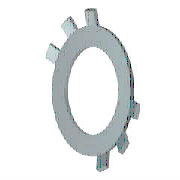
# Autodesk Inventor part: 垫圈 GB 858 30
Saved by Autodesk Inventor 2020 (Build 240168000, 168)
## iProperties
Created: 2019-01-21
Part Number: 垫圈 GB 858 30
Material: 钢，软
Description: 圆螺母的止动垫圈
Document SubType Name: Modeling
Standard: GB/T 858-1988
Designer: dell
Standard Revision: 1988
Standards Organization: GB
Language: zh-CN
Size Designation: 30 x 40
Categories: <MemberInstance><Categories><Category DisplayName="轴用零件" InternalName="7f7aeb1f-a693-4053-b835-cee3144e0d98" Mnemonic="SHFT"><Category DisplayName="止动垫圈" InternalName="196297a3-bbf2-4c62-a426-6f1b43e49a92" Mnemonic="STWRDBRCMP"><CategoryParameter DisplayName="接触区域直径" InternalName="2e92645a-023d-4b6f-85cb-aa6579b07711" Mnemonic="conarea"/><CategoryParameter DisplayName="沟槽高度" InternalName="459e1daf-c3a8-40cb-aa85-2a4675385d1b" Mnemonic="grvheig"/><CategoryParameter DisplayName="厚度" InternalName="5f8ad5cd-5310-44ac-8ee3-8a10cbe3cc2a" Mnemonic="thick"/><CategoryParameter DisplayName="轴直径" InternalName="a5cdae98-95ea-47ec-9880-d704d388e74c" Mnemonic="shaftdia"/></Category></Category><Category DisplayName="数据类型" InternalName="23b78d0f-2648-40c6-8793-ca6db495c9e8" Mnemonic="DATATYPE"><CategoryParameter DisplayName="显示名" InternalName="05415f3d-3907-474b-a020-eb9d644f4cf3" Mnemonic="DISPLAYNAME"/><CategoryParameter DisplayName="标准" InternalName="0c0a119c-1e12-4c84-803f-101930972f5e" Mnemonic="STANDARD"/><CategoryParameter DisplayName="描述" InternalName="13903e3d-64b1-4950-80da-f627842ea37f" Mnemonic="DESCRIPTION"/><CategoryParameter DisplayName="规格" InternalName="2675968c-4ce5-49e0-a4f5-552d29089031" Mnemonic="DESIGNATION"/><CategoryParameter DisplayName="默认列" InternalName="2af9ec52-faaa-4026-b378-f9fa4afca842" Mnemonic="DEFAULTROW"/><CategoryParameter DisplayName="文件夹名称" InternalName="3f06958e-8713-4116-9be7-ed6184ecc97b" Mnemonic="FOLDERNAME"/><CategoryParameter DisplayName="版本指南" InternalName="45a75005-10b1-4dfc-8d6d-dfe629f0b93c" Mnemonic="REVISIONGUID"/><CategoryParameter DisplayName="文件名" InternalName="8b46a4cc-9585-4fed-90c3-899f57e09a73" Mnemonic="FILENAME"/><CategoryParameter DisplayName="标准组织" InternalName="8f5914e1-4693-403f-8ab5-d37768198c9d" Mnemonic="STDSORG"/><CategoryParameter DisplayName="系列版本" InternalName="914462f6-6e19-4b14-ba84-155b9680b1d0" Mnemonic="FAMILYREVISION"/><CategoryParameter DisplayName="标准版本" InternalName="91d5a463-65c2-4fde-b823-3b7fea5e8e17" Mnemonic="STANDARDREVISION"/><CategoryParameter DisplayName="成员版本" InternalName="a65d44b9-392f-4f4f-857b-e4b3d54996fe" Mnemonic="MEMBERREVISION"/><CategoryParameter DisplayName="剪裁格式" InternalName="bc51e27b-3422-4e78-93ef-cec197ddf230" Mnemonic="CLIPFORMAT"/><CategoryParameter DisplayName="制造商" InternalName="cd6c7a72-a28a-4e50-99a9-2c7f4e13e5ad" Mnemonic="MANUFACTURER"/><CategoryParameter DisplayName="内部名称" InternalName="cf1d0246-76d9-4b4a-8305-fa0409afb5c1" Mnemonic="INTERNALNAME"/><CategoryParameter DisplayName="是否公制" InternalName="e2385c5b-1ea4-4823-96a8-8de651266ec3" Mnemonic="ISMETRIC"/><Category DisplayName="零件" InternalName="c0e0b642-3bcb-4cc8-9e80-f96d35c4afa4" Mnemonic="PART"><CategoryParameter DisplayName="零件代号" InternalName="016b6077-bfbe-49bd-92c9-d8d59c39c941" Mnemonic="PARTNUMBER"/><CategoryParameter DisplayName="库存编号" InternalName="4dba7c1c-e26c-444e-836c-b08b433409a8" Mnemonic="STOCKNUMBER"/><CategoryParameter DisplayName="材料键" InternalName="5c9a8adb-dd2b-4535-b97f-0a94a95fe41f" Mnemonic="MATERIALKEY"/><CategoryParameter DisplayName="材料" InternalName="818a152a-d3c3-49ca-80ee-df7d91421b8e" Mnemonic="MATERIAL"/></Category></Category><Category DisplayName="先前版本映射" InternalName="cd87c42b-3e48-431e-b5c0-1cbeb14dfe77" Mnemonic="LEGACYMAP"><CategoryParameter DisplayName="唯一 DA 成员 ID" InternalName="0918ad47-427f-4fed-ae26-24c81c58f590" Mnemonic="DACOOKIE"/><CategoryParameter DisplayName="合并11 ID" InternalName="0ee8fb18-e2ed-4f39-96f6-1f4b5f50aa71" Mnemonic="MERGE11"/><CategoryParameter DisplayName="唯一 CC 成员 ID" InternalName="5193edd4-b2b0-4ab4-9d54-de900eee34e0" Mnemonic="CCCOOKIE"/><CategoryParameter DisplayName="分割 ID" InternalName="72b5c83c-be7f-45c4-ae51-9160ea6deb26" Mnemonic="SPLIT"/><CategoryParameter DisplayName="成员 ID" InternalName="8e5e0294-fc51-4c8f-b3d7-003dc5ed94f6" Mnemonic="MEMBERID"/><CategoryParameter DisplayName="目录名" InternalName="d99d1e27-aa94-4de2-af4c-c348882a6f4f" Mnemonic="CATALOGNAME"/><CategoryParameter DisplayName="系列编号" InternalName="e705e1f4-09cb-413e-91f9-551b4188271e" Mnemonic="FAMILYNUMBER"/></Category></Categories><FamilyTemplate Id="wa1000"><FamilyTemplateParameters><FamilyTemplateParameter ObjectType="kUserParameterObject" ValueType="xs:double" Id="1" ObjectReferenceKey="SEWI"/><FamilyTemplateParameter ObjectType="kUserParameterObject" ValueType="xs:double" Id="2" ObjectReferenceKey="SD"/><FamilyTemplateParameter ObjectType="kUserParameterObject" ValueType="xs:double" Id="3" ObjectReferenceKey="RR"/><FamilyTemplateParameter ObjectType="kUserParameterObject" ValueType="xs:double" Id="4" ObjectReferenceKey="NND"/><FamilyTemplateParameter ObjectType="kUserParameterObject" ValueType="xs:double" Id="5" ObjectReferenceKey="ANG1"/><FamilyTemplateParameter ObjectType="kUserParameterObject" ValueType="xs:double" Id="6" ObjectReferenceKey="SD3"/><FamilyTemplateParameter ObjectType="kUserParameterObject" ValueType="xs:double" Id="7" ObjectReferenceKey="FAWI"/><FamilyTemplateParameter ObjectType="kUserParameterObject" ValueType="xs:double" Id="8" ObjectReferenceKey="PB"/><FamilyTemplateParameter ObjectType="kUserParameterObject" ValueType="xs:double" Id="9" ObjectReferenceKey="TL1"/><FamilyTemplateParameter ObjectType="kUserParameterObject" ValueType="xs:double" Id="10" ObjectReferenceKey="TW0"/><FamilyTemplateParameter ObjectType="kUserParameterObject" ValueType="xs:double" Id="11" ObjectReferenceKey="LADI"/><FamilyTemplateParameter ObjectType="kUserParameterObject" ValueType="xs:double" Id="12" ObjectReferenceKey="SD1"/><FamilyTemplateParameter ObjectType="kUserParameterObject" ValueType="xs:double" Id="13" ObjectReferenceKey="PNT"/><FamilyTemplateParameter ObjectType="kUserParameterObject" ValueType="xs:double" Id="14" ObjectReferenceKey="SD2"/><FamilyTemplateParameter ObjectType="kPropertyObject" ValueType="xs:string" Id="100" ObjectReferenceKey="{32853F0F-3444-11d1-9E93-0060B03C1CA6}" SubObjectId="52"/><FamilyTemplateParameter ObjectType="kPropertyObject" ValueType="xs:string" Id="105" ObjectReferenceKey="{32853F0F-3444-11d1-9E93-0060B03C1CA6}" SubObjectId="5"/><FamilyTemplateParameter ObjectType="kPartComponentDefinitionObject" ValueType="xs:string" Id="110" SubObjectId="Material"/></FamilyTemplateParameters></FamilyTemplate><CategoryParameterMap><ParamToTemplateMap><ParamToTemplate CategoryParameter="//CategoryParameter[@InternalName='05415f3d-3907-474b-a020-eb9d644f4cf3']" ConstantValue="Washer GB/T 858-1988"/><ParamToTemplate CategoryParameter="//CategoryParameter[@InternalName='cf1d0246-76d9-4b4a-8305-fa0409afb5c1']" ConstantValue="53e2c8ed-1660-418b-a02d-66a9e420a20d"/><ParamToTemplate CategoryParameter="//CategoryParameter[@InternalName='3f06958e-8713-4116-9be7-ed6184ecc97b']" ConstantValue="GB 858-88"/><ParamToTemplate CategoryParameter="//CategoryParameter[@InternalName='914462f6-6e19-4b14-ba84-155b9680b1d0']" ConstantValue="10"/><ParamToTemplate CategoryParameter="//CategoryParameter[@InternalName='bc51e27b-3422-4e78-93ef-cec197ddf230']" ConstantValue="CF_INVENTOR.STDPARTS"/><ParamToTemplate CategoryParameter="//CategoryParameter[@InternalName='e2385c5b-1ea4-4823-96a8-8de651266ec3']" ConstantValue="true"/><ParamToTemplate CategoryParameter="//CategoryParameter[@InternalName='13903e3d-64b1-4950-80da-f627842ea37f']" ConstantValue="Tab washers for round nut"/><ParamToTemplate CategoryParameter="//CategoryParameter[@InternalName='8f5914e1-4693-403f-8ab5-d37768198c9d']" ConstantValue="GB"/><ParamToTemplate CategoryParameter="//CategoryParameter[@InternalName='0c0a119c-1e12-4c84-803f-101930972f5e']" ConstantValue="GB/T 858-1988"/><ParamToTemplate CategoryParameter="//CategoryParameter[@InternalName='cd6c7a72-a28a-4e50-99a9-2c7f4e13e5ad']" TemplateParameter="104"/><ParamToTemplate CategoryParameter="//CategoryParameter[@InternalName='91d5a463-65c2-4fde-b823-3b7fea5e8e17']" ConstantValue="1988"/><ParamToTemplate CategoryParameter="//CategoryParameter[@InternalName='45a75005-10b1-4dfc-8d6d-dfe629f0b93c']" ConstantValue="f783c5b8-5933-49d5-a788-eb1b1bb6e0de"/><ParamToTemplate CategoryParameter="//CategoryParameter[@InternalName='2af9ec52-faaa-4026-b378-f9fa4afca842']" ConstantValue="10"/><ParamToTemplate CategoryParameter="//CategoryParameter[@InternalName='d99d1e27-aa94-4de2-af4c-c348882a6f4f']" ConstantValue="GB"/><ParamToTemplate CategoryParameter="//CategoryParameter[@InternalName='e705e1f4-09cb-413e-91f9-551b4188271e']" ConstantValue="309"/><ParamToTemplate CategoryParameter="//CategoryParameter[@InternalName='8b46a4cc-9585-4fed-90c3-899f57e09a73']" ConstantValue="垫圈 GB 858 30"/><ParamToTemplate CategoryParameter="//CategoryParameter[@InternalName='a65d44b9-392f-4f4f-857b-e4b3d54996fe']" ConstantValue="daddb7de-3eb2-4640-936e-600e5f022451"/><ParamToTemplate CategoryParameter="//CategoryParameter[@InternalName='8e5e0294-fc51-4c8f-b3d7-003dc5ed94f6']" ConstantValue="110"/><ParamToTemplate CategoryParameter="//CategoryParameter[@InternalName='2675968c-4ce5-49e0-a4f5-552d29089031']" TemplateParameter="100"/><ParamToTemplate CategoryParameter="//CategoryParameter[@InternalName='2e92645a-023d-4b6f-85cb-aa6579b07711']" TemplateParameter="11"/><ParamToTemplate CategoryParameter="//CategoryParameter[@InternalName='818a152a-d3c3-49ca-80ee-df7d91421b8e']" TemplateParameter="110"/><ParamToTemplate CategoryParameter="//CategoryParameter[@InternalName='a5cdae98-95ea-47ec-9880-d704d388e74c']" TemplateParameter="4"/><ParamToTemplate CategoryParameter="//CategoryParameter[@InternalName='016b6077-bfbe-49bd-92c9-d8d59c39c941']" TemplateParameter="105"/><ParamToTemplate CategoryParameter="//CategoryParameter[@InternalName='5f8ad5cd-5310-44ac-8ee3-8a10cbe3cc2a']" TemplateParameter="2"/></ParamToTemplateMap></CategoryParameterMap></MemberInstance>
Density: 7.85 g/cm^3
Appearance: 半抛光
_DisabledCommands: 0
IsCustomPart: 0
Author: dell
Autodesk Inventor part; units mm, degrees
ref_plane "YZ Plane" through (0, 0, 0) normal (1, 0, 0) x (0, 1, 0)
ref_plane "XZ Plane" through (0, 0, 0) normal (0, 1, 0) x (-1, 0, 0)
sketch "草图1" plane through (0, 0, 0) normal (0, 0, 1) x (1, 0, 0)
  line L0 (-0.580263, 0) -> (3.481577, 0)
  line L1 (0, 3.8) -> (0, 13.95)
  line L2 (0, 20.221695) -> (2.694468, 26)
  line L3 (2.694468, 26) -> (3.600776, 25.577382)
  line L4 (3.600776, 25.577382) -> (1, 20)
  line L5 (1, 20) -> (1, 15.25)
  line L6 (1, 15.25) -> (0, 15.25)
  dimension "d1" = 1
  dimension "d2" = 30.5
  dimension "d3" = 40
  dimension "d4" = 52
  dimension "d5" = 25
  dimension "d6" = 1
  constraints: 10 end point, 3 perpendicular, 2 point on line, 1 parallel
  measures "d1" distance between parallel lines of L4 L2
  measures "d2" diameter of L6 L0
  measures "d3" diameter of L4.end L0
  measures "d4" diameter of L2.end L0
  measures "d5" angle of L1 L2
  measures "d6" distance between parallel lines of L1 L5
sketch "草图1 outline for 轴承体" plane through (0, 0, 0) normal (0, 0, 1) x (1, 0, 0)
  line L0 (2.694468, 26) -> (0, 20.221695)
  line L1 (3.600776, 25.577382) -> (2.694468, 26)
  line L2 (1, 20) -> (3.600776, 25.577382)
  line L3 (1, 15.25) -> (1, 20)
  line L4 (0, 15.25) -> (1, 15.25)
  line L5 (0, 20.221695) -> (0, 15.25)
revolve "轴承体" add sketch "草图1 outline for 轴承体" angle 360 about axis through (-10, 0, 0) along (1, 0, 0)
sketch "草图2" plane through (0, 0, 0) normal (-1, 0, 0) x (0, 0, 1)
  line L0 (0, -36.4) -> (0, 36.4)
  line L1 (2.4, 15.059963) -> (2.4, 11.75)
  line L2 (2.4, 11.75) -> (0, 11.75)
  line L3 (-2.4, 15.059963) -> (-2.4, 11.75)
  line L4 (-2.4, 11.75) -> (0, 11.75)
  line L5 (-36.4, 0) -> (36.4, 0)
  circle A0 centre (0, 0) radius 15.25
  circle A1 centre (0, 0) radius 26
  circle A2 centre (0, 0) radius 20
  line L6 (-2.4, 12.75) -> (2.4, 12.75)
  circle A3 centre (0, 0) radius 20.221695
  line L7 (2.4, 19.855478) -> (2.4, 25.888994)
  line L8 (0, 36.4) -> (0, -36.4)
  line L9 (0, 0) -> (13, 22.51666) construction
  line L10 (7.849278, 18.395348) -> (10.866036, 23.620526)
  line L11 (12.0062, 15.995348) -> (15.022958, 21.220526)
  line L12 (-2.4, 19.855478) -> (-2.4, 25.888994)
  line L13 (0, 0) -> (22.51666, 13) construction
  line L14 (15.995348, 12.0062) -> (21.220526, 15.022958)
  line L15 (18.395348, 7.849278) -> (23.620526, 10.866036)
  line L16 (0, 0) -> (-25.114071, -6.729295) construction
  line L17 (-19.800085, -2.820754) -> (-25.628013, -4.382343)
  line L18 (-18.557753, -7.457198) -> (-24.385682, -9.018787)
  line L19 (0, 0) -> (-18.384776, -18.384776) construction
  line L20 (0, 0) -> (-6.729295, -25.114071) construction
  line L21 (-15.736999, -12.342887) -> (-20.003339, -16.609227)
  line L22 (-12.342887, -15.736999) -> (-16.609227, -20.003339)
  line L23 (-7.457198, -18.557753) -> (-9.018787, -24.385682)
  line L24 (-2.820754, -19.800085) -> (-4.382343, -25.628013)
  dimension "d9" = 4.8
  dimension "d21" = 1
  dimension "d25" = 27
  dimension "d32" = 4.8
  dimension "d34" = 4.8
  dimension "d36" = 30
  dimension "d38" = 2.4
  dimension "d39" = 30
  dimension "d40" = 15
  dimension "d41" = 4.8
  dimension "d42" = 30
  dimension "d43" = 30
  dimension "d45" = 4.8
  dimension "d47" = 4.8
  constraints: 44 end point, 5 parallel, 4 point on line, 2 midpoint, 2 perpendicular, 2 point on circle, 2 vertical alignment, 1 symmetric about line, 39 other
  measures "d9" diameter of L1 L0
  measures "d21" distance between parallel lines of L2 L6
  measures "d32" distance between parallel lines of L11 L10
  measures "d34" distance between parallel lines of L15 L14
  measures "d36" angle of L8 L9
  measures "d38" distance between parallel lines of L8 L3
  measures "d39" angle of L9 L13
  measures "d40" angle of L16 L5
  measures "d41" distance between parallel lines of L18 L17
  measures "d42" angle of L19 L16
  measures "d43" angle of L20 L19
  measures "d45" distance between parallel lines of L22 L21
  measures "d47" distance between parallel lines of L24 L23
sketch "草图2 outline for 切口" plane through (0, 0, 0) normal (-1, 0, 0) x (0, 0, 1)
  arc A0 (-7.457198, -18.557753) -> (-12.342887, -15.736999) centre (0, 0) cw
  line L0 (-9.018787, -24.385682) -> (-7.457198, -18.557753)
  arc A1 (-16.609227, -20.003339) -> (-9.018787, -24.385682) centre (0, 0) ccw
  line L1 (-12.342887, -15.736999) -> (-16.609227, -20.003339)
  arc A2 (-15.736999, -12.342887) -> (-18.557753, -7.457198) centre (0, 0) cw
  line L2 (-20.003339, -16.609227) -> (-15.736999, -12.342887)
  arc A3 (-24.385682, -9.018787) -> (-20.003339, -16.609227) centre (0, 0) ccw
  line L3 (-18.557753, -7.457198) -> (-24.385682, -9.018787)
  line L4 (2.4, 25.888994) -> (2.4, 19.855478)
  arc A4 (10.866036, 23.620526) -> (2.4, 25.888994) centre (0, 0) ccw
  line L5 (7.849278, 18.395348) -> (10.866036, 23.620526)
  arc A5 (2.4, 19.855478) -> (7.849278, 18.395348) centre (0, 0) cw
  line L6 (15.022958, 21.220526) -> (12.0062, 15.995348)
  arc A6 (21.220526, 15.022958) -> (15.022958, 21.220526) centre (0, 0) ccw
  line L7 (15.995348, 12.0062) -> (21.220526, 15.022958)
  arc A7 (12.0062, 15.995348) -> (15.995348, 12.0062) centre (0, 0) cw
  arc A8 (-19.800085, -2.820754) -> (-2.4, 19.855478) centre (0, 0) cw
  line L8 (-25.628013, -4.382343) -> (-19.800085, -2.820754)
  arc A9 (-2.4, 25.888994) -> (-25.628013, -4.382343) centre (0, 0) ccw
  line L9 (-2.4, 19.855478) -> (-2.4, 25.888994)
  line L10 (23.620526, 10.866036) -> (18.395348, 7.849278)
  arc A10 (-4.382343, -25.628013) -> (23.620526, 10.866036) centre (0, 0) ccw
  line L11 (-2.820754, -19.800085) -> (-4.382343, -25.628013)
  arc A11 (18.395348, 7.849278) -> (-2.820754, -19.800085) centre (0, 0) cw
extrude "切口" cut sketch "草图2 outline for 切口" against normal through all
extrude "榫1" add sketch "草图2" against normal blind 1 contours L4 L3 L6 L0 | L0 L6 L1 L2 | A0 L0 L6 L3 | L1 L6 L0 A0
extrude "榫2" add sketch "草图2" against normal blind 5 contours L4 L3 L6 L0 | L0 L6 L1 L2
ref_plane "Work Plane1" through (0.5, 0, 0) normal (0, 0, -1) x (1, 0, 0)
equation "\"d1\" = SD"
equation "\"d2\" = SD1"
equation "\"d3\" = LADI"
equation "\"d4\" = SD2"
equation "\"d5\" = FAWI"
equation "\"d6\" = SD"
equation "\"d9\" = TW0"
equation "\"d21\" = SD"
equation "\"d25\" = SD3"
equation "\"d32\" = TW0"
equation "\"d34\" = TW0"
equation "\"d36\" = SEWI"
equation "\"d39\" = SEWI"
equation "\"d40\" = ANG1"
equation "\"d41\" = TW0"
equation "\"d42\" = SEWI"
equation "\"d43\" = SEWI"
equation "\"d45\" = TW0"
equation "\"d47\" = TW0"
equation "\"d17\" = SD"
equation "\"d13\" = SD"
equation "\"d23\" = TL1"
equation "\"FAWI\" = 25deg"
equation "\"SD1\" = 30.5"
equation "\"SD2\" = 52"
equation "\"SD\" = 1"
equation "\"TW0\" = 4.8"
equation "\"LADI\" = 40"
equation "\"d8\" = SD1"
equation "\"TL1\" = 5"
equation "\"SD3\" = 27"
equation "\"SEWI\" = 30deg"
equation "\"ANG1\" = 15deg"
equation "\"RR\" = 0.1"
equation "\"PB\" = TW0"
equation "\"PNT\" = TL1"
body "Solid1"
